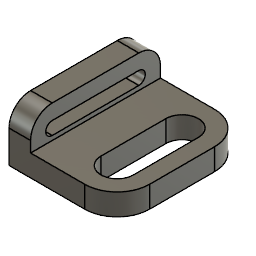
Exercise_2 (Autodesk Fusion 360 design; units mm, degrees)
part number: 2026-05-18-22-52-03-926
Autodesk Fusion 360 part; units mm, degrees
sketch "Sketch1" plane through (0, 0, 0) normal (0, 1, 0) x (1, 0, 0)
  line L0 (50, 60) -> (-50, 60)
  line L1 (-50, 60) -> (-50, -60)
  line L2 (-50, -60) -> (50, -60)
  line L3 (50, -60) -> (50, 60)
  line L4 (50, 60) -> (-50, -60) construction
  line L5 (-50, 60) -> (50, -60) construction
  line L6 (50, -60) -> (20, -60)
  line L7 (20, -60) -> (20, -30)
  line L8 (50, 60) -> (20, 60)
  line L9 (20, 60) -> (20, 30)
  line L10 (35, 30) -> (35, -30)
  line L11 (5, 30) -> (5, -30)
  arc A0 (35, 30) -> (5, 30) centre (20, 30) ccw
  arc A1 (5, -30) -> (35, -30) centre (20, -30) ccw
  line L12 (-50, -60) -> (-30, -60)
  line L13 (-30, -60) -> (-30, 60)
  line L14 (-30, 60) -> (-50, 60)
  dimension "d1" = 100
  dimension "d2" = 120
  dimension "d3" = 30
  dimension "d4" = 30
  dimension "d5" = 30
  dimension "d6" = 30
  dimension "d7" = 30
  dimension "d8" = 30
  dimension "d9" = 20
  constraint horizontal L0
  constraint perpendicular L0 L1
  constraint parallel L0 L2
  constraint parallel L1 L3
  constraint coincident L4 origin
  constraint coincident L5 origin
  constraint perpendicular L3 L6
  constraint perpendicular L6 L7
  constraint coincident L7.end A1.centre
  constraint perpendicular L3 L8
  constraint perpendicular L8 L9
  constraint coincident L9.end A0.centre
  constraint tangent L10 A1
  constraint parallel L3 L10
  constraint tangent L11 A1
  constraint parallel L10 L11
  constraint perpendicular L1 L12
  constraint coincident L0 L13.end
  constraint perpendicular L0 L13
  measures "d1" distance of L1.end L2.end
  measures "d2" distance of L0.end L1.end
  measures "d3" distance of L2.end L6.end
  measures "d4" distance of L6.end L7.end
  measures "d5" diameter of A1
  measures "d6" distance of L0.start L8.end
  measures "d7" distance of L8.end L9.end
  measures "d8" diameter of A0
  measures "d9" distance of L1.end L12.end
extrude "Extrude1" add sketch "Sketch1" along normal blind 20 contours L0 L2 L3 L6 L7 L8 L9 L10 A0 A1 | L0 L2 L7 L9 L11 A0 A1 L13
extrude "Extrude2" add sketch "Sketch1" along normal blind 50 contours L0 L1 L2 L12 L13 L14
sketch "Sketch2" plane through (-30, 0, 0) normal (1, 0, 0) x (0, 0, -1)
  line L0 (-60, 20) -> (60, 20)
  line L1 (60, 20) -> (60, 50)
  line L2 (60, 50) -> (-60, 50)
  line L3 (-60, 50) -> (-60, 20)
  line L4 (-40, 36) -> (-40, 30)
  line L5 (40, 36) -> (40, 30)
  line L6 (-40, 36) -> (40, 36)
  line L7 (40, 24) -> (-40, 24)
  arc A0 (-40, 36) -> (-40, 24) centre (-40, 30) ccw
  arc A1 (40, 24) -> (40, 36) centre (40, 30) ccw
  dimension "d16" = 12
  dimension "d19" = 12
  constraint coincident L4.end A0.centre
  constraint coincident L5.end A1.centre
  constraint tangent L7 A0
  constraint parallel L0 L7
  measures "d16" diameter of A0
  measures "d19" diameter of A1
extrude "Extrude3" cut sketch "Sketch2" against normal blind 20 contours L6 L7 A0 A1
fillet "Fillet1" radius 20 2 edges at (-40, 50, 60) (-40, 50, -60)
fillet "Fillet1" radius 30 2 edges at (50, 10, 60) (50, 10, -60)
